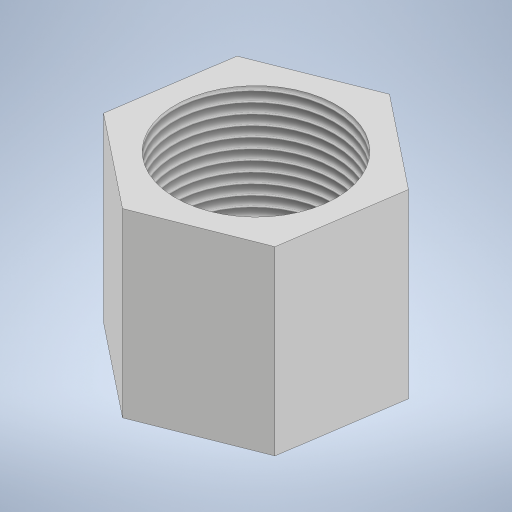
# Autodesk Inventor part: HUDSON1--43
Saved by Autodesk Inventor 2024.2 (Build 282272000, 272)
## iProperties
Created: 2024-10-10
Part Number: HUDSON1--43
Material: Generic
Document SubType Name: Modeling
Designer: Precisión-05
Density: 1 g/cm^3
Appearance: Default
Author: Precisión-05
Autodesk Inventor part; units mm, degrees
ref_plane "YZ Plane" through (0, 0, 0) normal (1, 0, 0) x (0, 1, 0)
ref_plane "XZ Plane" through (0, 0, 0) normal (0, 1, 0) x (-1, 0, 0)
ref_plane "XY Plane" through (0, 0, 0) normal (0, 0, 1) x (1, 0, 0)
sketch "Sketch1" plane through (0, 0, 0) normal (0, 0, 1) x (1, 0, 0)
  line L0 (1.7136, 11.547) -> (10.8568, 4.2894)
  line L1 (10.8568, 4.2894) -> (9.1432, -7.2576)
  line L2 (9.1432, -7.2576) -> (-1.7136, -11.547)
  line L3 (-1.7136, -11.547) -> (-10.8568, -4.2894)
  line L4 (-10.8568, -4.2894) -> (-9.1432, 7.2576)
  line L5 (-9.1432, 7.2576) -> (1.7136, 11.547)
  point P0 (0, 0)
  point P1 (0, 0)
  dimension "d0" = 20
  constraints: 12 end point, 1 coincident, 13 other
  measures "d0" horizontal distance of L0.end L4.end
extrude "Extrusion1" add sketch "Sketch1" along normal blind 18
sketch "Sketch2" plane through (0, 0, 18) normal (0, 0, 1) x (1, 0, 0)
  point P0 (0, 0)
  point P1 (0, 0)
  constraints: 1 coincident
hole "Hole1" at (0, 0, 18) direction (0, 0, -1) diameter 11 depth 18 counterbore diameter 16 counterbore depth 14
thread "Thread1" size "M16x1" class "6H" standard "ANSI Metric M Profile" full length
body "Solid1"
